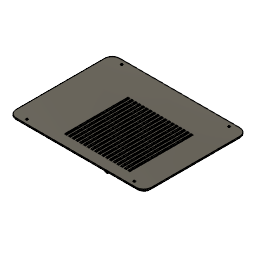
Mini PC Lid V3 (Autodesk Fusion 360 design; units mm, degrees)
Autodesk Fusion 360 part; units mm, degrees
note: some values were not read from the file. Set by a fixed rule: which sketch regions a step uses.
sketch "Sketch1" plane through (0, 0, 0) normal (0, 0, 1) x (1, 0, 0)
  line L0 (10, 0) -> (200, 0)
  line L1 (210, 10) -> (210, 150)
  line L2 (200, 160) -> (10, 160)
  line L3 (0, 150) -> (0, 10)
  arc A0 (10, 160) -> (0, 150) centre (10, 150) ccw
  arc A1 (210, 150) -> (200, 160) centre (200, 150) ccw
  arc A2 (200, 0) -> (210, 10) centre (200, 10) ccw
  arc A3 (0, 10) -> (10, 0) centre (10, 10) ccw
  line L4 (200, 162) -> (10, 162)
  arc A4 (10, 162) -> (-2, 150) centre (10, 150) ccw
  line L5 (-2, 150) -> (-2, 10)
  arc A5 (-2, 10) -> (10, -2) centre (10, 10) ccw
  line L6 (10, -2) -> (200, -2)
  arc A6 (200, -2) -> (212, 10) centre (200, 10) ccw
  line L7 (212, 10) -> (212, 150)
  arc A7 (212, 150) -> (200, 162) centre (200, 150) ccw
  line L8 (200, 155) -> (10, 155)
  arc A8 (10, 155) -> (5, 150) centre (10, 150) ccw
  line L9 (5, 150) -> (5, 10)
  arc A9 (5, 10) -> (10, 5) centre (10, 10) ccw
  line L10 (10, 5) -> (200, 5)
  arc A10 (200, 5) -> (205, 10) centre (200, 10) ccw
  line L11 (205, 10) -> (205, 150)
  arc A11 (205, 150) -> (200, 155) centre (200, 150) ccw
  circle A12 centre (20, 5) radius 1.1
  circle A13 centre (20, 5) radius 3
  circle A14 centre (60, 85) radius 1.1
  circle A15 centre (180, 76) radius 1.1
  circle A16 centre (144, 9) radius 1.1
  circle A17 centre (144, 9) radius 3
  circle A18 centre (60, 85) radius 3
  circle A19 centre (180, 76) radius 3
  line L12 (105, 162) -> (105, -2) construction
  line L13 (212, 80) -> (-2, 80) construction
  circle A20 centre (190, 5) radius 3
  circle A21 centre (190, 5) radius 1.1
  circle A22 centre (20, 155) radius 3
  circle A23 centre (20, 155) radius 1.1
  circle A24 centre (190, 155) radius 3
  circle A25 centre (190, 155) radius 1.1
  point P0 (210, 0)
  point P1 (0, 160)
  dimension "d1" = 210
  dimension "d2" = 160
  dimension "d4" = 10
  dimension "d5" = 2
  dimension "d6" = -5
  dimension "d9" = 2.2
  dimension "d10" = 6
  dimension "d11" = 20
  dimension "d12" = 5
  dimension "d13" = 2.2
  dimension "d14" = 2.2
  dimension "d15" = 2.2
  dimension "d17" = 75
  dimension "d18" = 84
  dimension "d19" = 30
  dimension "d21" = 66
  dimension "d22" = 9
  dimension "d23" = 60
  dimension "d24" = 6
  dimension "d25" = 6
  dimension "d26" = 6
  dimension "d31" = 170
  dimension "d32" = 150
  constraint horizontal L0
  constraint vertical L1
  constraint horizontal L2
  constraint vertical L3
  constraint coincident P1 L2
  constraint coincident P1 L3
  constraint tangent L2 A0
  constraint tangent L3 A0
  constraint tangent L1 A1
  constraint tangent L2 A1
  constraint equal A0 A1
  constraint coincident P0 L0
  constraint coincident P0 L1
  constraint tangent L0 A2
  constraint tangent L1 A2
  constraint equal A0 A2
  constraint coincident origin L0
  constraint coincident origin L3
  constraint tangent L0 A3
  constraint tangent L3 A3
  constraint equal A0 A3
  constraint concentric A12 A13
  constraint concentric A16 A17
  constraint concentric A14 A18
  constraint concentric A15 A19
  constraint midpoint L4 L12.start
  constraint midpoint L6 L12.end
  constraint midpoint L7 L13.start
  constraint midpoint L5 L13.end
  measures "d1" distance of origin P0
  measures "d2" distance of origin P1
  measures "d4" radius of A0
  measures "d9" diameter of A12
  measures "d10" diameter of A13
  measures "d11" distance of L3 A12.centre
  measures "d12" distance of L0 A12.centre
  measures "d13" diameter of A14
  measures "d14" diameter of A15
  measures "d15" diameter of A16
  measures "d17" distance of L2 A14.centre
  measures "d18" distance of L2 A15.centre
  measures "d19" distance of L1 A15.centre
  measures "d21" distance of L1 A16.centre
  measures "d22" distance of L0 A16.centre
  measures "d23" distance of L3 A14.centre
  measures "d24" diameter of A17
  measures "d25" diameter of A18
  measures "d26" diameter of A19
extrude "Extrude1" add sketch "Sketch1" against normal blind 1 contours L0 L1 L2 L3 A0 A1 A2 A3 | L4 A4 L5 A5 L6 A6 L7 A7 | L8 A8 L9 A9 L10 A10 L11 A11 A13 A20 A22 A24 | L8 A24 A25 | L8 A24 A25 | L8 A25 | L8 A25 | L8 A22 A23 | L8 A22 A23 | L8 A23 | L8 A23 | L10 A20 A21 | L10 A20 A21 | L10 A21 | L10 A21 | L10 A12 A13 | L10 A12 A13 | L10 A12 | L10 A12 | A14 | A15 | A16 | A17 | A18 | A19
extrude "Extrude2" add sketch "Sketch1" against normal blind 3 contours L0 L1 L2 L3 A0 A1 A2 A3 | L8 A24 A25 | L8 A24 A25 | L8 A22 A23 | L8 A22 A23 | L10 A20 A21 | L10 A20 A21 | L10 A12 A13 | L10 A12 A13 | A17 | A18 | A19
sketch "Sketch3" plane through (0, 0, -1) normal (0, 0, -1) x (1, 0, 0)
  arc A0 (200, -162) -> (212, -150) centre (200, -150) ccw
  line L0 (212, -150) -> (212, -10)
  arc A1 (212, -10) -> (200, 2) centre (200, -10) ccw
  line L1 (200, 2) -> (10, 2)
  arc A2 (10, 2) -> (-2, -10) centre (10, -10) ccw
  line L2 (-2, -10) -> (-2, -150)
  arc A3 (-2, -150) -> (10, -162) centre (10, -150) ccw
  line L3 (10, -162) -> (200, -162)
  circle A4 centre (190, -155) radius 2.25
  circle A5 centre (20, -155) radius 2.25
  circle A6 centre (66, -85) radius 2.25
  circle A7 centre (186, -76) radius 2.25
  circle A8 centre (190, -5) radius 2.25
  circle A9 centre (150, -9) radius 2.25
  circle A10 centre (20, -5) radius 2.25
  line L4 (10, 0) -> (200, 0)
  arc A11 (210, -10) -> (200, 0) centre (200, -10) ccw
  line L5 (210, -10) -> (210, -150)
  arc A12 (200, -160) -> (210, -150) centre (200, -150) ccw
  line L6 (200, -160) -> (10, -160)
  arc A13 (0, -150) -> (10, -160) centre (10, -150) ccw
  line L7 (0, -150) -> (0, -10)
  arc A14 (10, 0) -> (0, -10) centre (10, -10) ccw
  dimension "d38" = 4.5
  dimension "d39" = 4.5
  dimension "d40" = 4.5
  dimension "d41" = 4.5
  dimension "d42" = 4.5
  dimension "d43" = 4.5
  dimension "d44" = 4.5
  measures "d38" diameter of A4
  measures "d39" diameter of A5
  measures "d40" diameter of A6
  measures "d41" diameter of A7
  measures "d42" diameter of A8
  measures "d43" diameter of A9
  measures "d44" diameter of A10
extrude "Extrude5" cut 4 faces at (189.4633, 4.7506, -1) (20.2286, 5.396, -1) (20.2286, 154.7133, -1) (189.8112, 154.6587, -1) along direction (0, 0, -1) up to surface end surface through (0, 0, 0) normal (0, 0, 1) offset 0
extrude "Extrude6" add 3 faces at (178.3747, 74.2886, -3) (146.3555, 8.851, -3) (62.0302, 83.7962, -3) along direction (0, 0, -1) blind 8
chamfer "Chamfer2" distance 2 angle 45 3 edges at (177.203, 74.9152, -1) (141.203, 7.9152, -1) (57.203, 83.9152, -1)
sketch "Sketch4" plane through (0, 0, -1) normal (0, 0, -1) x (1, 0, 0)
  circle A0 centre (180, -76) radius 5
  arc A1 (141, -5) -> (147, -5) centre (144, -9) ccw
  line L0 (141, -5) -> (23, -5)
  arc A2 (17, -5) -> (23, -5) centre (20, -5) ccw
  line L1 (17, -5) -> (10, -5)
  arc A3 (10, -5) -> (5, -10) centre (10, -10) ccw
  line L2 (5, -10) -> (5, -150)
  arc A4 (5, -150) -> (10, -155) centre (10, -150) ccw
  line L3 (10, -155) -> (17, -155)
  arc A5 (23, -155) -> (17, -155) centre (20, -155) ccw
  line L4 (23, -155) -> (187, -155)
  arc A6 (193, -155) -> (187, -155) centre (190, -155) ccw
  line L5 (193, -155) -> (200, -155)
  arc A7 (200, -155) -> (205, -150) centre (200, -150) ccw
  line L6 (205, -150) -> (205, -10)
  arc A8 (205, -10) -> (200, -5) centre (200, -10) ccw
  line L7 (200, -5) -> (193, -5)
  arc A9 (187, -5) -> (193, -5) centre (190, -5) ccw
  line L8 (187, -5) -> (147, -5)
  circle A10 centre (60, -85) radius 5
  line L9 (70, -115) -> (73, -115)
  line L10 (73, -115) -> (73, -15)
  line L11 (73, -15) -> (70, -15)
  line L12 (70, -15) -> (70, -115)
  line L13 (75.8824, -15) -> (75.8824, -115)
  line L14 (75.8824, -115) -> (78.8824, -115)
  line L15 (78.8824, -115) -> (78.8824, -15)
  line L16 (78.8824, -15) -> (75.8824, -15)
  line L17 (81.7647, -15) -> (81.7647, -115)
  line L18 (81.7647, -115) -> (84.7647, -115)
  line L19 (84.7647, -115) -> (84.7647, -15)
  line L20 (84.7647, -15) -> (81.7647, -15)
  line L21 (87.6471, -15) -> (87.6471, -115)
  line L22 (87.6471, -115) -> (90.6471, -115)
  line L23 (90.6471, -115) -> (90.6471, -15)
  line L24 (90.6471, -15) -> (87.6471, -15)
  line L25 (93.5294, -15) -> (93.5294, -115)
  line L26 (93.5294, -115) -> (96.5294, -115)
  line L27 (96.5294, -115) -> (96.5294, -15)
  line L28 (96.5294, -15) -> (93.5294, -15)
  line L29 (99.4118, -15) -> (99.4118, -115)
  line L30 (99.4118, -115) -> (102.4118, -115)
  line L31 (102.4118, -115) -> (102.4118, -15)
  line L32 (102.4118, -15) -> (99.4118, -15)
  line L33 (105.2941, -15) -> (105.2941, -115)
  line L34 (105.2941, -115) -> (108.2941, -115)
  line L35 (108.2941, -115) -> (108.2941, -15)
  line L36 (108.2941, -15) -> (105.2941, -15)
  line L37 (111.1765, -15) -> (111.1765, -115)
  line L38 (111.1765, -115) -> (114.1765, -115)
  line L39 (114.1765, -115) -> (114.1765, -15)
  line L40 (114.1765, -15) -> (111.1765, -15)
  line L41 (117.0588, -15) -> (117.0588, -115)
  line L42 (117.0588, -115) -> (120.0588, -115)
  line L43 (120.0588, -115) -> (120.0588, -15)
  line L44 (120.0588, -15) -> (117.0588, -15)
  line L45 (122.9412, -15) -> (122.9412, -115)
  line L46 (122.9412, -115) -> (125.9412, -115)
  line L47 (125.9412, -115) -> (125.9412, -15)
  line L48 (125.9412, -15) -> (122.9412, -15)
  line L49 (128.8235, -15) -> (128.8235, -115)
  line L50 (128.8235, -115) -> (131.8235, -115)
  line L51 (131.8235, -115) -> (131.8235, -15)
  line L52 (131.8235, -15) -> (128.8235, -15)
  line L53 (134.7059, -15) -> (134.7059, -115)
  line L54 (134.7059, -115) -> (137.7059, -115)
  line L55 (137.7059, -115) -> (137.7059, -15)
  line L56 (137.7059, -15) -> (134.7059, -15)
  line L57 (140.5882, -15) -> (140.5882, -115)
  line L58 (140.5882, -115) -> (143.5882, -115)
  line L59 (143.5882, -115) -> (143.5882, -15)
  line L60 (143.5882, -15) -> (140.5882, -15)
  line L61 (146.4706, -15) -> (146.4706, -115)
  line L62 (146.4706, -115) -> (149.4706, -115)
  line L63 (149.4706, -115) -> (149.4706, -15)
  line L64 (149.4706, -15) -> (146.4706, -15)
  line L65 (152.3529, -15) -> (152.3529, -115)
  line L66 (152.3529, -115) -> (155.3529, -115)
  line L67 (155.3529, -115) -> (155.3529, -15)
  line L68 (155.3529, -15) -> (152.3529, -15)
  line L69 (158.2353, -15) -> (158.2353, -115)
  line L70 (158.2353, -115) -> (161.2353, -115)
  line L71 (161.2353, -115) -> (161.2353, -15)
  line L72 (161.2353, -15) -> (158.2353, -15)
  line L73 (164.1176, -15) -> (164.1176, -115)
  line L74 (164.1176, -115) -> (167.1176, -115)
  line L75 (167.1176, -115) -> (167.1176, -15)
  line L76 (167.1176, -15) -> (164.1176, -15)
  line L77 (170, -15) -> (170, -115)
  line L78 (170, -115) -> (173, -115)
  line L79 (173, -115) -> (173, -15)
  line L80 (173, -15) -> (170, -15)
  dimension "d53" = 3
  dimension "d54" = 100
  dimension "d69" = 100
  dimension "d70" = 0
  constraint horizontal L9
  constraint vertical L10
  constraint horizontal L11
  constraint vertical L12
  measures "d53" distance of L9.start L9.end
  measures "d54" distance of L9.start L11.end
extrude "Extrude7" cut sketch "Sketch4" against normal blind 2 contours L9 L10 L11 L12 | L13 L14 L15 L16 | L17 L18 L19 L20 | L21 L22 L23 L24 | L25 L26 L27 L28 | L29 L30 L31 L32 | L33 L34 L35 L36 | L37 L38 L39 L40 | L41 L42 L43 L44 | L45 L46 L47 L48 | L49 L50 L51 L52 | L53 L54 L55 L56 | L57 L58 L59 L60 | L61 L62 L63 L64 | L65 L66 L67 L68 | L69 L70 L71 L72 | L73 L74 L75 L76 | L77 L78 L79 L80
extrude "Extrude9" add 1 faces at (178.3747, 74.2886, -11) along direction (0, 0, -1) blind 2
extrude "Extrude10" add 1 faces at (62.0302, 83.7962, -11) along direction (0, 0, -1) blind 1
extrude "Extrude11" add 1 faces at (22, 91.6667, 0) along direction (0, 0, 1) blind 1
chamfer "Chamfer3" distance 0.5 angle 45 4 edges at (188.9744, 155.3978, 1) (18.9744, 155.3978, 1) (18.9744, 5.3978, 1) (188.9744, 5.3978, 1)
equation "BoxRadius = 10 mm"
equation "d4 = BoxRadius"
equation "HolesRadius = 2.2 mm"
equation "HolesOuterRadius = 6 mm"
equation "d9 = HolesRadius"
equation "d10 = HolesOuterRadius"
equation "d13 = HolesRadius"
equation "d14 = HolesRadius"
equation "d15 = HolesRadius"
equation "d24 = HolesOuterRadius"
equation "d25 = HolesOuterRadius"
equation "d26 = HolesOuterRadius"
equation "BoltHead = 4.5 mm"
equation "d38 = BoltHead"
equation "d39 = BoltHead"
equation "d40 = BoltHead"
equation "d41 = BoltHead"
equation "d42 = BoltHead"
equation "d43 = BoltHead"
equation "d44 = BoltHead"
